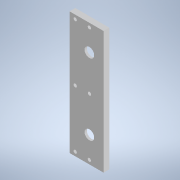
# Autodesk Inventor part: pi_cam_stereo_case_cover
Saved by Autodesk Inventor 2021 (Build 250183000, 183)
## iProperties
Created: 2020-12-07
Part Number: pi_cam_stereo_case_cover
Material: Generic
Document SubType Name: Modeling
Designer: Mateusz
Density: 1 g/cm^3
Appearance: Default
Author: Mateusz
Autodesk Inventor part; units mm, degrees
ref_plane "YZ Plane" through (0, 0, 0) normal (1, 0, 0) x (0, 1, 0)
ref_plane "XZ Plane" through (0, 0, 0) normal (0, 1, 0) x (-1, 0, 0)
ref_plane "Work Plane1" through (0, 0, 0) normal (0, 0, 1) x (1, 0, 0)
sketch "Sketch1" plane through (0, 0, 0) normal (0, 0, 1) x (1, 0, 0)
  line L0 (-12.431, 44.25) -> (12.431, 44.25) projected
  line L1 (12.431, 44.25) -> (12.431, -44.25) projected
  line L2 (12.431, -44.25) -> (-12.431, -44.25) projected
  line L3 (-12.431, -44.25) -> (-12.431, 44.25) projected
  line L4 (-14.931, 46.75) -> (-14.931, -46.75) projected
  line L5 (-14.931, -46.75) -> (14.931, -46.75) projected
  line L6 (14.931, -46.75) -> (14.931, 46.75) projected
  line L7 (14.931, 46.75) -> (-14.931, 46.75) projected
  circle A0 centre (-9.931, -20.75) radius 1.1 projected
  circle A1 centre (-9.931, -41.75) radius 1.1 projected
  circle A2 centre (2.569, -41.75) radius 1.1 projected
  circle A3 centre (2.569, -20.75) radius 1.1 projected
  circle A4 centre (-9.931, 20.75) radius 1.1 projected
  circle A5 centre (2.569, 20.75) radius 1.1 projected
  circle A6 centre (-9.931, 41.75) radius 1.1 projected
  circle A7 centre (2.569, 41.75) radius 1.1 projected
  line L8 (6.4721, 35.2583) -> (-1.5279, 35.2583) projected
  line L9 (-1.5279, 35.2583) -> (-1.5279, 27.2583) projected
  line L10 (-1.5279, 27.2583) -> (6.4721, 27.2583) projected
  line L11 (6.4721, 27.2583) -> (6.4721, 35.2583) projected
  circle A8 centre (2.4721, 31.2583) radius 3.8 projected
  line L12 (6.4721, -27.2417) -> (-1.5279, -27.2417) projected
  line L13 (-1.5279, -27.2417) -> (-1.5279, -35.2417) projected
  line L14 (-1.5279, -35.2417) -> (6.4721, -35.2417) projected
  line L15 (6.4721, -35.2417) -> (6.4721, -27.2417) projected
  circle A9 centre (2.4721, -31.2417) radius 3.8 projected
  point P0 (0, 0)
extrude "Extrusion1" add sketch "Sketch1" along normal blind 2 contours L0 L1 L2 L3 | L7 L6 L5 L4
sketch "Sketch2" plane through (0, 0, 2) normal (0, 0, 1) x (1, 0, 0)
  line L0 (-1.5279, 27.2583) -> (6.4721, 27.2583) projected
  line L1 (-1.5279, 35.2583) -> (-1.5279, 27.2583) projected
  line L2 (6.4721, 35.2583) -> (-1.5279, 35.2583) projected
  line L3 (6.4721, 27.2583) -> (6.4721, 35.2583) projected
  line L4 (-1.5279, -27.2417) -> (-1.5279, -35.2417) projected
  line L5 (-1.5279, -35.2417) -> (6.4721, -35.2417) projected
  line L6 (6.4721, -27.2417) -> (-1.5279, -27.2417) projected
  line L7 (6.4721, -35.2417) -> (6.4721, -27.2417) projected
  line L8 (6.4721, -35.2417) -> (-1.5279, -35.2417) projected
  line L9 (-1.5279, -35.2417) -> (-1.5279, -35.4417)
  line L10 (-1.5279, -35.4417) -> (6.4721, -35.4417)
  line L11 (6.4721, -35.4417) -> (6.6721, -35.4417)
  line L12 (6.6721, -35.4417) -> (6.6721, -27.2417)
  line L13 (6.6721, -27.2417) -> (6.6721, -27.0417)
  line L14 (6.6721, -27.0417) -> (-1.5279, -27.0417)
  line L15 (-1.5279, -27.0417) -> (-1.7279, -27.0417)
  line L16 (-1.7279, -27.0417) -> (-1.7279, -35.4417)
  line L17 (-1.7279, -35.4417) -> (-1.5279, -35.4417)
  line L18 (6.4721, 35.2583) -> (6.4721, 27.2583) projected
  line L19 (6.4721, 27.2583) -> (6.6721, 27.2583)
  line L20 (6.6721, 27.2583) -> (6.6721, 35.2583)
  line L21 (6.6721, 35.2583) -> (6.6721, 35.4583)
  line L22 (6.6721, 35.4583) -> (-1.5279, 35.4583)
  line L23 (-1.5279, 35.4583) -> (-1.7279, 35.4583)
  line L24 (-1.7279, 35.4583) -> (-1.7279, 27.2583)
  line L25 (-1.7279, 27.2583) -> (-1.7279, 27.0583)
  line L26 (-1.7279, 27.0583) -> (6.6721, 27.0583)
  line L27 (6.6721, 27.0583) -> (6.6721, 27.2583)
  point P0 (0, 0)
  dimension "d2" = 0.2
  dimension "d3" = 0.2
  dimension "d4" = 0.2
  dimension "d5" = 0.2
  dimension "d6" = 0.2
  dimension "d7" = 0.2
  dimension "d8" = 0.2
  dimension "d9" = 0.2
  constraints: 36 end point, 14 point on line, 6 perpendicular, 1 parallel, 1 vertical
  measures "d2" distance of L4.end L9.end
  measures "d3" distance of L10.end L11.end
  measures "d4" distance of L12.end L13.end
  measures "d5" distance of L14.end L15.end
  measures "d6" distance of L0.end L19.end
  measures "d7" distance of L20.end L21.end
  measures "d8" distance of L22.end L23.end
  measures "d9" distance of L24.end L25.end
extrude "Extrusion2" cut sketch "Sketch2" against normal through all
sketch "Sketch3" plane through (0, 0, 0) normal (0, 0, -1) x (-1, 0, 0)
  line L0 (12.431, 44.25) -> (-12.431, 44.25) projected
  line L1 (-12.431, 44.25) -> (-12.431, -44.25) projected
  line L2 (-12.431, -44.25) -> (12.431, -44.25) projected
  line L3 (12.431, -44.25) -> (12.431, 44.25) projected
  line L4 (14.931, 46.75) -> (14.931, -46.75) projected
  line L5 (14.931, -46.75) -> (-14.931, -46.75) projected
  line L6 (-14.931, -46.75) -> (-14.931, 46.75) projected
  line L7 (-14.931, 46.75) -> (14.931, 46.75) projected
  point P0 (0, 0)
extrude "Extrusion3" add sketch "Sketch3" along normal blind 3.05
sketch "Sketch4" plane through (0, 0, 2) normal (0, 0, 1) x (1, 0, 0)
  line L0 (6.6721, -35.4417) -> (-1.7279, -35.4417) projected
  line L1 (-1.7279, -35.4417) -> (-1.7279, -27.0417) projected
  line L2 (-1.7279, -27.0417) -> (6.6721, -27.0417) projected
  line L3 (6.6721, -27.0417) -> (6.6721, -35.4417) projected
  line L4 (-1.7279, 27.0583) -> (-1.7279, 35.4583) projected
  line L5 (6.6721, 27.0583) -> (-1.7279, 27.0583) projected
  line L6 (6.719, 35.5) -> (-1.781, 35.5) projected
  line L7 (6.6721, 35.4583) -> (6.6721, 27.0583) projected
  line L8 (6.6721, 27.0583) -> (6.6721, 35.4583) projected
  line L9 (6.6721, 31.2583) -> (2.4721, 31.2583)
  line L10 (-1.7279, 27.0583) -> (6.6721, 27.0583) projected
  line L11 (2.4721, 31.2583) -> (2.4721, 35.4583)
  line L12 (6.6721, 35.4583) -> (-1.7279, 35.4583) projected
  line L13 (6.6721, -31.2417) -> (2.4721, -31.2417)
  line L14 (2.4721, -31.2417) -> (2.4721, -27.0417)
  circle A0 centre (2.4721, 31.2583) radius 4.2
  circle A1 centre (2.4721, -31.2417) radius 4.2
  point P0 (0, 0)
  point P1 (2.4721, -35.4417)
  point P2 (-1.7279, -31.2417)
  point P3 (-1.7279, 31.2583)
  point P4 (2.4721, 27.0583)
  constraints: 8 end point, 4 midpoint, 2 coincident, 1 parallel, 1 perpendicular, 1 point on line, 6 other
extrude "Extrusion4" add sketch "Sketch4" against normal up to surface (2 mm away) contours L0 A1 L3 | L0 L1 A1 | A1 L2 L3 | L1 L2 A1 | L4 A0 L5 | L4 L12 A0 | A0 L7 L5 | L12 L7 A0
sketch "Sketch5" plane through (0, 0, 0) normal (0, 0, -1) x (-1, 0, 0)
  circle A0 centre (9.931, -20.75) radius 2 projected
  circle A1 centre (9.931, -41.75) radius 2 projected
  circle A2 centre (-2.569, -41.75) radius 2 projected
  circle A3 centre (-2.569, -20.75) radius 2 projected
  circle A4 centre (9.931, 20.75) radius 2 projected
  circle A5 centre (-2.569, 20.75) radius 2 projected
  circle A6 centre (9.931, 41.75) radius 2 projected
  circle A7 centre (-2.569, 41.75) radius 2 projected
  circle A8 centre (-2.569, 20.75) radius 1.1 projected
  circle A9 centre (9.931, 20.75) radius 1.1 projected
  circle A10 centre (9.931, 41.75) radius 1.1 projected
  circle A11 centre (-2.569, 41.75) radius 1.1 projected
  circle A12 centre (9.931, -20.75) radius 1.1 projected
  circle A13 centre (-2.569, -20.75) radius 1.1 projected
  circle A14 centre (-2.569, -41.75) radius 1.1 projected
  circle A15 centre (9.931, -41.75) radius 1.1 projected
  point P0 (0, 0)
extrude "Extrusion5" add sketch "Sketch5" along normal blind 3.05
sketch "Sketch6" plane through (0, 0, 2) normal (0, 0, 1) x (1, 0, 0)
  circle A0 centre (-9.931, -20.75) radius 1.1 projected
  line L0 (-9.931, -20.75) -> (-9.931, 0)
  circle A1 centre (-9.931, 0) radius 1.45
  circle A2 centre (2.569, 0) radius 1.45
  circle A3 centre (-9.931, 0) radius 3
  circle A4 centre (2.569, 0) radius 3
  point P0 (0, 0)
  dimension "d18" = 20.75
  dimension "d19" = 2.9
  dimension "d20" = 2.9
  dimension "d21" = 6
  dimension "d22" = 6
  constraints: 4 centre point, 3 coincident, 2 end point, 1 vertical
  measures "d18" distance of L0.start L0.end
  measures "d19" diameter of A1
  measures "d20" diameter of A2
  measures "d21" diameter of A3
  measures "d22" diameter of A4
extrude "Extrusion6" cut sketch "Sketch6" against normal through all contours A1 | A2
extrude "Extrusion7" add sketch "Sketch6" against normal up to surface (5.05 mm away) contours A3 | A4
sketch "Sketch7" plane through (0, 0, 2) normal (0, 0, 1) x (1, 0, 0)
  circle A0 centre (2.569, 20.75) radius 1.1 projected
  circle A1 centre (-9.931, 20.75) radius 1.1 projected
  circle A2 centre (2.569, 41.75) radius 1.1 projected
  circle A3 centre (-9.931, 41.75) radius 1.1 projected
  circle A4 centre (2.569, -20.75) radius 1.1 projected
  circle A5 centre (2.569, -41.75) radius 1.1 projected
  circle A6 centre (-9.931, -41.75) radius 1.1 projected
  circle A7 centre (-9.931, -20.75) radius 1.1 projected
  point P0 (0, 0)
extrude "Extrusion8" add sketch "Sketch7" against normal up to surface (5.05 mm away)
sketch "Sketch8" plane through (2.569, -41.75, -3.05) normal (0, 0, -1) x (-1, 0, 0)
  circle A0 centre (0, 0) radius 2 projected
  circle A1 centre (0, 0) radius 0.8
  circle A2 centre (12.5, 0) radius 2 projected
  circle A3 centre (12.5, 0) radius 0.8
  circle A4 centre (12.5, 21) radius 2 projected
  circle A5 centre (12.5, 21) radius 0.8
  circle A6 centre (0, 21) radius 2 projected
  circle A7 centre (0, 21) radius 0.8
  circle A8 centre (0, 62.5) radius 2 projected
  circle A9 centre (0, 62.5) radius 0.8
  circle A10 centre (12.5, 62.5) radius 2 projected
  circle A11 centre (12.5, 62.5) radius 0.8
  circle A12 centre (12.5, 83.5) radius 2 projected
  circle A13 centre (12.5, 83.5) radius 0.8
  circle A14 centre (0, 83.5) radius 2 projected
  circle A15 centre (0, 83.5) radius 0.8
  point P0 (2.569, 41.75)
  dimension "d29" = 1.6
  dimension "d30" = 1.6
  dimension "d31" = 1.6
  dimension "d32" = 1.6
  dimension "d33" = 1.6
  dimension "d34" = 1.6
  dimension "d35" = 1.6
  dimension "d36" = 1.6
  constraints: 8 centre point, 8 coincident
  measures "d29" diameter of A1
  measures "d30" diameter of A3
  measures "d31" diameter of A5
  measures "d32" diameter of A7
  measures "d33" diameter of A9
  measures "d34" diameter of A11
  measures "d35" diameter of A13
  measures "d36" diameter of A15
extrude "Extrusion9" add sketch "Sketch8" along normal blind 1 contours A1 | A3 | A5 | A7 | A9 | A11 | A13 | A15
sketch "Sketch9" plane through (0, 0, 2) normal (0, 0, 1) x (1, 0, 0)
  circle A0 centre (-9.931, -50.25) radius 1.45 projected
  circle A1 centre (2.473, -50.25) radius 1.45 projected
  circle A2 centre (-9.931, 50.25) radius 1.45 projected
  circle A3 centre (2.473, 50.25) radius 1.45 projected
  line L0 (-12.431, 44.25) -> (12.431, 44.25) projected
  line L1 (12.431, 44.25) -> (12.431, -44.25) projected
  line L2 (12.431, -44.25) -> (-12.431, -44.25) projected
  line L3 (-12.431, -44.25) -> (-12.431, 44.25) projected
  line L4 (-14.931, -53.75) -> (-14.931, 53.75) projected
  line L5 (14.931, -53.75) -> (-14.931, -53.75) projected
  line L6 (14.931, 53.75) -> (14.931, -53.75) projected
  line L7 (-14.931, 53.75) -> (14.931, 53.75) projected
  point P0 (0, 0)
extrude "Extrusion10" add sketch "Sketch9" against normal up to surface (5.05 mm away)
body "Solid1"
